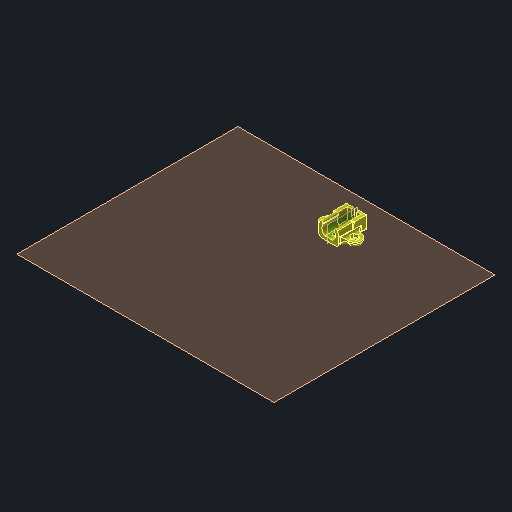
# Autodesk Inventor part: MScIR_WingedMotorHolder-tightened
Saved by Autodesk Inventor 2026.1 (Build 301233020, 233B)
## iProperties
Created: 2018-10-10
Part Number: MScIR_WingedMotorHolder-tightened
Material: ABS Plastic
Document SubType Name: Modeling
Designer: mja502
Density: 1.06 g/cm^3
Appearance: Smooth - White
mountWingsHoleSpacing: 25,200 mm
Author: mja502
Autodesk Inventor part; units mm, degrees
ref_plane "YZ Plane" through (0, 0, 0) normal (1, 0, 0) x (0, 1, 0)
sketch "Body  Clip Bulk OL" plane through (0, 0, 0) normal (0, 0, 1) x (1, 0, 0)
  line L0 (-3.5, 3) -> (3.5, 3)
  line L1 (0, 0) -> (0, 19.508) construction
  line L2 (-6, 8) -> (6, 8) construction
  line L3 (-3.5, 13) -> (3.5, 13)
  arc A0 (-3.5, 13) -> (-3.5, 3) centre (0.25, 8) ccw
  arc A1 (3.5, 3) -> (3.5, 13) centre (-0.25, 8) ccw
  line L4 (4.3935, 16) -> (-4.3935, 16)
  arc A2 (-4.3935, 16) -> (-9, 8) centre (0.25, 8) ccw
  arc A3 (9, 8) -> (4.3935, 16) centre (-0.25, 8) ccw
  line L5 (-9, 8) -> (-9, 0)
  line L6 (9, 8) -> (9, 0)
  line L7 (-9, 0) -> (9, 0)
  point P0 (0, 0)
  point P1 (0, 3)
  point P2 (0, 8)
  point P3 (0, 13)
  point P4 (0, 16)
  dimension "d1" = 7
  dimension "d3" = 12
  dimension "d4" = 5
  dimension "d5" = 10
  dimension "d6" = 3
  dimension "d8" = 3
  dimension "d9" = 18
  constraints: 16 end point, 10 point on circle, 5 midpoint, 4 centre point, 4 horizontal, 4 point on line, 3 vertical, 1 coincident, 1 parallel, 1 tangent
  measures "d1" distance of L0.start L0.end
  measures "d3" distance of L2.start L2.end
  measures "d4" distance between parallel lines of L0 L2
  measures "d5" distance between parallel lines of L0 L3
  measures "d6" distance between parallel lines of L3 L4
  measures "d8" distance from line of point (0, 0) L0
  measures "d9" distance of L5.end L6.end
extrude "Body Clip Bulk" add sketch "Body  Clip Bulk OL" along normal blind 13.8
fillet "Clip Bottom Fillet" radius 2 2 edges at (-9, 0, 6.9) (9, 0, 6.9)
ref_plane "BC Midplane" through (-3.5, 8, 0) normal (0, 1, 0) x (1, 0, 0)
sketch "BC Top Cut OL" plane through (0.0033, 16, 0) normal (0, 1, 0) x (-1, 0, 0)
  line L0 (-5.1967, 13.8) -> (5.2033, 13.8)
  line L1 (5.2033, 13.8) -> (5.2033, 0)
  line L2 (5.2033, 0) -> (-5.1967, 0)
  line L3 (-5.1967, 0) -> (-5.1967, 13.8)
  point P0 (0.0033, 0)
  point P1 (0.0033, 0)
  dimension "d13" = 10.4
  dimension "d14" = 13.8
  constraints: 8 end point, 2 parallel, 1 coincident, 1 horizontal, 1 midpoint, 1 perpendicular
  measures "d13" distance of L0.start L0.end
  measures "d14" distance of L0.end L1.end
extrude "BC Top Cut" cut sketch "BC Top Cut OL" against normal up to surface (8 mm away)
fillet "BC Top Edge Fillets" radius 1.4 2 edges at (5.2, 15.474, 6.9) (-5.2, 15.474, 6.9)
sketch "BC Removal Slot OL" plane through (-3.5, 3, 0) normal (0, 1, 0) x (1, 0, 0)
  line L0 (3.5, 0) -> (3.5, -13.8) construction
  line L1 (7, -13.8) -> (0, -13.8) construction
  line L2 (7, 0) -> (7, -13.8) construction
  line L3 (7, -6.9) -> (0, -6.9) construction
  line L4 (0, 0) -> (0, -13.8) construction
  line L5 (3.5, -5.9) -> (3.5, -7.9) construction
  line L6 (1.5, -5.9) -> (1.5, -7.9)
  line L7 (5.5, -7.9) -> (5.5, -5.9)
  arc A0 (5.5, -5.9) -> (1.5, -5.9) centre (3.5, -5.9) ccw
  arc A1 (1.5, -7.9) -> (5.5, -7.9) centre (3.5, -7.9) ccw
  point P0 (3.5, -6.9)
  dimension "d79" = 6
  dimension "d80" = 4
  constraints: 12 end point, 5 midpoint, 4 point on circle, 4 tangent, 2 centre point, 1 parallel, 1 point on line
  measures "d80" distance between parallel lines of L6 L7
extrude "BC Removal Slot" cut sketch "BC Removal Slot OL" against normal through all
sketch "FS Floor Bulk OL" plane through (0, 0, 0) normal (0, 0, 1) x (1, 0, 0)
  line L0 (-9, 0) -> (9, 0)
  line L1 (9, 0) -> (9, 2.6)
  line L2 (9, 2.6) -> (-9, 2.6)
  line L3 (-9, 2.6) -> (-9, 0)
  line L4 (-7, 0) -> (7, 0) projected
  point P0 (0, 0)
  point P1 (0, 0)
  dimension "d19" = 18
  dimension "d20" = 2.6
  constraints: 8 end point, 2 midpoint, 2 parallel, 1 horizontal, 1 perpendicular
  measures "d19" distance of L0.start L0.end
  measures "d20" distance of L2.end L0.start
extrude "FS Floor Bulk" add sketch "FS Floor Bulk OL" against normal blind 11.2
fillet "FS Bottom Fillet" radius 3 2 edges at (9, 0, -5.6) (-9, 0, -5.6)
sketch "FS Walls OL" plane through (-3.5, 2.6, 4.5) normal (0, 1, 0) x (1, 0, 0)
  line L0 (3.5, 4.5) -> (3.5, 19.7596) construction
  line L1 (-5.5, 4.5) -> (-2.5, 4.5)
  line L2 (-2.5, 4.5) -> (-2.5, 13.7)
  line L3 (-2.5, 13.7) -> (1.3, 13.7)
  line L4 (1.3, 13.7) -> (1.3, 15.7)
  line L5 (1.3, 15.7) -> (-5.5, 15.7)
  line L6 (-5.5, 15.7) -> (-5.5, 4.5)
  line L7 (12.5, 4.5) -> (9.5, 4.5)
  line L8 (9.5, 4.5) -> (9.5, 13.7)
  line L9 (9.5, 13.7) -> (5.7, 13.7)
  line L10 (5.7, 13.7) -> (5.7, 15.7)
  line L11 (5.7, 15.7) -> (12.5, 15.7)
  line L12 (12.5, 15.7) -> (12.5, 4.5)
  dimension "d24" = 6.8
  dimension "d25" = 2
  dimension "d26" = 3
  dimension "d27" = 9.2
  dimension "d28" = 11.2
  dimension "d32" = 9
  constraints: 26 end point, 6 symmetric about line, 5 perpendicular, 1 horizontal, 1 vertical
  measures "d24" distance of L4.end L5.end
  measures "d25" distance of L3.end L4.end
  measures "d26" distance of L1.start L1.end
  measures "d27" distance of L1.end L2.end
  measures "d28" vertical distance of L0.start L5.end
  measures "d32" distance of L0.start L1.start
extrude "FS Walls" add sketch "FS Walls OL" along normal blind 10.4
sketch "FS Shaft Slot Seat OL" plane through (0, 0, -11.2) normal (0, 0, -1) x (-1, 0, 0)
  line L0 (0, 0) -> (0, 7.8) construction
  circle A0 centre (0, 7.8) radius 2.2
  line L1 (-2.2, 7.8) -> (-2.2, 2.6)
  line L2 (-2.2, 2.6) -> (2.2, 2.6)
  line L3 (2.2, 2.6) -> (2.2, 7.8)
  dimension "d33" = 7.8
  dimension "d34" = 4.4
  dimension "d35" = 5.2
  dimension "d36" = 4.4
  constraints: 8 end point, 2 coincident, 2 perpendicular, 2 point on circle, 2 vertical, 1 centre point, 1 parallel
  measures "d33" distance of L0.start L0.end
  measures "d34" diameter of A0
  measures "d35" distance of L2.end L3.end
  measures "d36" distance of L1.end L2.end
extrude "FS Front Shaft Seat" add sketch "FS Shaft Slot Seat OL" against normal blind 2 contours L3 L2 L1 A0
sketch "FS Pillars OL" plane through (-3.5, 3, 13.8) normal (0, 1, 0) x (1, 0, 0)
  line L0 (8.9, 13.8) -> (9.5, 13.8)
  line L1 (9.5, 13.8) -> (9.5, 15.7)
  line L2 (9.5, 15.7) -> (8.9, 15.7)
  line L3 (8.9, 15.7) -> (8.9, 13.8)
  line L4 (-2.5, 16.1) -> (-1.9, 16.1)
  line L5 (-1.9, 16.1) -> (-1.9, 20)
  line L6 (-1.9, 20) -> (-2.5, 20)
  line L7 (-2.5, 20) -> (-2.5, 16.1)
  point P0 (3.5, 13.8)
  dimension "d39" = 0.6
  dimension "d40" = 1.9
  dimension "d41" = 6
  dimension "d42" = 0
  dimension "d43" = 0.6
  dimension "d44" = 3.9
  dimension "d46" = 6
  dimension "d47" = 2.3
  constraints: 16 end point, 4 parallel, 2 horizontal, 2 perpendicular
  measures "d39" distance of L2.end L1.end
  measures "d40" distance of L1.end L0.end
  measures "d41" distance of point (3.5, 13.8) L0.end
  measures "d42" distance from line of point (3.5, 13.8) L0
  measures "d43" distance of L6.end L5.end
  measures "d44" distance of L5.end L4.end
  measures "d46" horizontal distance of point (3.5, 13.8) L4.start
  measures "d47" distance from line of point (3.5, 13.8) L4
extrude "FS Pillars" [suppressed]
sketch "Sketch9" plane through (9, 8, 13.8) normal (1, 0, 0) x (0, 0, -1)
  line L0 (13.8, -6) -> (13.8, -5.4) projected
  line L1 (13.8, -5.4) -> (3.1659, 5.2341)
  line L2 (13.8, 5.2341) -> (0, 5.2341) projected
  line L3 (13.8, -5.4) -> (28.8388, -5.4) construction
  line L4 (13.8, -5.4) -> (13.8, 5.2341)
  point P0 (13.8, -8)
  dimension "d50" = 135
  constraints: 6 end point, 1 equal length, 1 horizontal, 1 point on line
  measures "d50" angle of L3 L1
extrude "BC 45deg cut" [suppressed]
ref_plane "Encoder Section Plane" through (0, 0, 13.8) normal (0, 0, 1) x (1, 0, 0)
sketch "Sketch10" plane through (0, 0, 13.8) normal (0, 0, 1) x (1, 0, 0)
  line L0 (-9, 2) -> (9, 2)
  line L1 (9, 2) -> (9, 0)
  line L2 (9, 0) -> (-9, 0)
  line L3 (-9, 0) -> (-9, 2)
  point P0 (0, 0)
  point P1 (0, 0)
  dimension "d54" = 2
  dimension "d55" = 18
  constraints: 8 end point, 2 parallel, 1 coincident, 1 horizontal, 1 midpoint, 1 perpendicular
  measures "d54" distance of L0.end L1.end
  measures "d55" distance of L1.end L2.end
extrude "ES Floor" [suppressed]
fillet "ES Bottom Fillet" [suppressed]
sketch "ES walls OL" plane through (-8.8284, 2, 13.8) normal (0, 1, 0) x (1, 0, 0)
  line L0 (-0.1716, 0) -> (-0.1716, -9.1)
  line L1 (-0.1716, -9.1) -> (17.8284, -9.1)
  line L2 (17.8284, -9.1) -> (17.8284, 0)
  line L3 (17.8284, 0) -> (15.5284, 0)
  line L4 (15.5284, 0) -> (15.5284, -7.1)
  line L5 (15.5284, -7.1) -> (2.1284, -7.1)
  line L6 (2.1284, -7.1) -> (2.1284, 0)
  line L7 (2.1284, 0) -> (-0.1716, 0)
  point P0 (8.8284, 13.8)
  dimension "d59" = 2.3
  dimension "d60" = 2
  dimension "d61" = 9.1
  dimension "d62" = 18
  constraints: 16 end point, 6 perpendicular, 2 equal length, 1 coincident, 1 horizontal, 1 point on line, 1 vertical
  measures "d59" distance between parallel lines of L2 L4
  measures "d60" distance between parallel lines of L1 L5
  measures "d61" distance of L1.end L2.end
  measures "d62" distance of L0.end L1.end
extrude "ES Walls" [suppressed]
sketch "ES Slot ol" plane through (-6.7, 2, 13.8) normal (0, 1, 0) x (1, 0, 0)
  line L0 (13.6, -1.8) -> (-0.2, -1.8)
  line L1 (-0.2, -1.8) -> (-0.2, -5.2)
  line L2 (-0.2, -5.2) -> (13.6, -5.2)
  line L3 (13.6, -5.2) -> (13.6, -1.8)
  line L4 (10.2, 0) -> (3.2, 0) construction
  line L5 (6.7, 0) -> (6.7, -5.8979) construction
  line L6 (13.6, -3.5) -> (-0.2, -3.5) construction
  point P0 (6.7, 13.8)
  point P1 (6.7, -1.8)
  dimension "d65" = 13.8
  dimension "d66" = 3.4
  dimension "d67" = 3.5
  constraints: 12 end point, 4 midpoint, 2 parallel, 1 horizontal, 1 perpendicular, 1 point on line, 1 vertical
  measures "d65" distance of L1.end L2.end
  measures "d66" distance of L0.end L1.end
  measures "d67" distance between parallel lines of L4 L6
extrude "ES Slot" [suppressed]
sketch "Sketch13" plane through (0, 0, 22.9) normal (0, 0, 1) x (1, 0, 0)
  line L0 (0, 0) -> (0, 7) construction
  line L1 (-6.1716, 0) -> (6.1716, 0) construction
  circle A0 centre (0, 7) radius 4.45
  line L2 (4.45, 7) -> (4.45, 13)
  line L3 (4.45, 13) -> (-4.45, 13)
  line L4 (-9, 13) -> (9, 13) construction
  line L5 (-4.45, 13) -> (-4.45, 7)
  point P0 (0, 0)
  dimension "d70" = 7
  dimension "d71" = 8.9
  constraints: 8 end point, 3 vertical, 2 point on circle, 2 tangent, 1 centre point, 1 coincident, 1 collinear, 1 midpoint, 1 perpendicular
  measures "d70" distance of L0.start L0.end
  measures "d71" diameter of A0
extrude "ES Rear Cutaway" [suppressed]
fillet "ES Merge Fillet" radius 0.95 4 edges at (-7.627, 12.7855, 0) (-8.7006, 10.3345, 0) (7.627, 12.7855, 0) (8.7006, 10.3345, 0)
fillet "ES Cutaway Fille" [suppressed]
sketch "Sketch16" plane through (-6.7, 2, 15.6) normal (0, 0, 1) x (1, 0, 0)
  arc A0 (-0.2, -1.9102) -> (0.5284, -2) centre (0.5284, 1) ccw projected
  line L0 (12.8716, -2) -> (0.5284, -2) projected
  arc A1 (12.8716, -2) -> (13.6, -1.9102) centre (12.8716, 1) ccw projected
  line L1 (13.6, 11) -> (13.6, -1.9102) projected
  line L2 (13.4, 11) -> (13.6, 11) projected
  line L3 (13.4, 0) -> (13.4, 11) projected
  line L4 (0, 0) -> (13.4, 0) projected
  line L5 (0, 11) -> (0, 0) projected
  line L6 (-0.2, 11) -> (0, 11) projected
  line L7 (-0.2, -1.9102) -> (-0.2, 11) projected
  point P0 (6.7, -2)
  point P1 (0, -1.9531)
  point P2 (13.4, -1.9531)
  constraints: 2 point on circle
extrude "ES Pins Undercut" [suppressed]
chamfer "ES Pins Undercut CHamfer" [suppressed]
ref_plane "Midplane" through (0, 0, 2.8) normal (0, 0, -1) x (-1, 0, 0)
sketch "Sketch17" plane through (-6, 0, -11.2) normal (0, -1, 0) x (1, 0, 0)
  line L0 (26.68, 14) -> (-18.68, 14) construction
  line L1 (6, 14) -> (6, 11.2) construction
  circle A0 centre (18.6, 14) radius 1.6 construction
  circle A1 centre (-6.6, 14) radius 1.6
  line L2 (-6.6, 8.4) -> (-6.6, 19.6) construction
  line L3 (-6.6, 14) -> (-12.2, 14) construction
  line L4 (-3, 0) -> (-3, 11.2) construction
  line L5 (-3, 25) -> (-3, 34.1) construction
  arc A2 (-6.6, 19.6) -> (-6.6, 8.4) centre (-6.6, 14) ccw
  arc A3 (-3, 4.8) -> (-6.6, 8.4) centre (-6.6, 4.8) ccw
  arc A4 (-6.6, 19.6) -> (-3, 23.2) centre (-6.6, 23.2) ccw
  line L6 (-3, 4.8) -> (-3, 23.2)
  dimension "d88" = 3.2
  dimension "d89" = 25.2
  dimension "d90" = 11.2
  dimension "d91" = 5.6
  constraints: 8 end point, 7 point on circle, 5 centre point, 5 point on line, 4 tangent, 3 vertical, 1 equal radius, 1 horizontal, 1 midpoint, 1 symmetric about line
  measures "d88" diameter of A0
  measures "d89" distance of L3.start A0.centre
  measures "d90" distance of L2.start L2.end
  measures "d91" distance of L3.start L3.end
extrude "Wing Bulk" add sketch "Sketch17" against normal blind 4.4
sketch "Sketch18" plane through (-9, 0, 12) normal (1, 0, 0) x (0, 0, -1)
  line L0 (0, 3) -> (12, 3) projected
  line L1 (0, 0) -> (0, 3) projected
  line L2 (0, 0) -> (18.4, 0) projected
  line L3 (18.4, 0) -> (18.4, 2.6) projected
  line L4 (18.4, 2.6) -> (12, 2.6) projected
  line L5 (12, 2.6) -> (12, 3) projected
  point P0 (12, 0)
extrude "Wing Underside Merge" add sketch "Sketch18" along normal up to surface (7 mm away)
fillet "Wing UNderside Fillet" radius 3 3 edges at (-18.2, 0, 2.8) (-10.0544, 0, -3.8544) (-10.0544, 0, 9.4544)
sketch "Sketch19" plane through (-6, 4.4, -11.2) normal (0, 1, 0) x (1, 0, 0)
  circle A0 centre (-6.6, -14) radius 1.6 projected
  line L0 (-6.6, -10.6514) -> (-3.7, -12.3257)
  line L1 (-3.7, -12.3257) -> (-3.7, -15.6743)
  line L2 (-3.7, -15.6743) -> (-6.6, -17.3486)
  line L3 (-6.6, -17.3486) -> (-9.5, -15.6743)
  line L4 (-9.5, -15.6743) -> (-9.5, -12.3257)
  line L5 (-9.5, -12.3257) -> (-6.6, -10.6514)
  line L6 (-17.6406, -14) -> (20.4437, -14) construction
  point P0 (6, -11.2)
  dimension "d98" = 5.8
  constraints: 12 end point, 1 coincident, 1 perpendicular, 13 other
  measures "d98" distance between parallel lines of L4 L1
extrude "Wing Nut Cut" cut sketch "Sketch19" against normal blind 2.4
mirror "Wing Mirror" about plane through (0, 0, 0) normal (1, 0, 0) of "Wing Bulk", "Wing Underside Merge", "Wing UNderside Fillet", "Wing Nut Cut"
fillet "Wings Top Fillet" radius 3 2 edges at (-9, 4.4, 2.8) (9, 4.4, 2.8)
sketch "Sketch20" plane through (6.7, 2, 19) normal (0, 0, -1) x (-1, 0, 0)
  line L0 (-0.2, 11) -> (-0.0716, 11) projected
  line L1 (-0.2, -1.9102) -> (-0.2, 11) projected
  arc A0 (-0.2, -1.9102) -> (0.5284, -2) centre (0.5284, 1) ccw projected
  line L2 (12.8716, -2) -> (0.5284, -2) projected
  arc A1 (12.8716, -2) -> (13.6, -1.9102) centre (12.8716, 1) ccw projected
  line L3 (13.6, -1.9102) -> (13.6, 11) projected
  line L4 (13.4716, 11) -> (13.6, 11) projected
  line L5 (13.4, 0) -> (13.4, 10.9995) projected
  line L6 (0, 0) -> (13.4, 0) projected
  line L7 (0, 10.9995) -> (0, 0) projected
  point P0 (6.7, -2)
  constraints: 2 other
extrude "Slot Enlarging" [suppressed]
sketch "Sketch21" plane through (-6, 0, 13.8) normal (0, -1, 0) x (1, 0, 0)
  arc A0 (4, -7.9) -> (8, -7.9) centre (6, -7.9) ccw projected
  line L0 (8, -5.9) -> (8, -7.9) projected
  arc A1 (8, -5.9) -> (4, -5.9) centre (6, -5.9) ccw projected
  line L1 (4, -7.9) -> (4, -5.9) projected
  point P0 (6, -13.8)
extrude "Extrusion18" cut sketch "Sketch21" against normal through all
ref_plane "Work Plane5" through (0, 2.6, -9.2) normal (-1, 0, 0) x (0, 0, 1)
ref_plane "Work Plane6" through (-15.0139, 0, 63.8653) normal (0, 1, 0) x (-1, 0, 0)
equation "\"d1\" = mo_mBodyFlatsWidth + mo_bcFlatWidthExtra"
equation "\"d3\" = mo_mBodyDiam + mo_bcBodyExtra"
equation "\"d4\" = 0.5 * mo_bcHeightExtra + 0.5 * mo_mBodyFlatsDiam"
equation "\"d5\" = mo_mBodyFlatsDiam + mo_bcHeightExtra"
equation "\"d6\" = mo_bcWallThickness"
equation "\"d8\" = mo_bcWallThickness"
equation "\"d9\" = mo_bcTotalWidth"
equation "\"d10\" = mo_bcLength"
equation "\"d12\" = mo_bcBottomFillet"
equation "\"d13\" = mo_bcTopCutWidth"
equation "\"d14\" = mo_bcLength"
equation "\"d15\" = mo_mBodyLength"
equation "\"d18\" = mo_bcOpeningFillet"
equation "\"d19\" = mo_fsTotalWidth"
equation "\"d20\" = mo_fsFloorDepth"
equation "\"d23\" = mo_fsBottomFillet"
equation "\"d24\" = 0.5 * mo_fsTotalWidth - 0.5 * mo_fsShaftSlotWidth"
equation "\"d25\" = mo_fsFrontThickness"
equation "\"d26\" = mo_fsWallThickness"
equation "\"d32\" = 0.5 * mo_fsTotalWidth"
equation "\"d30\" = mo_fsTotalHeight - mo_fsFloorDepth"
equation "\"d33\" = 0.5 * mo_mGbHeight + mo_fsFloorDepth + 0.5 * mo_fsShaftSlotClearance"
equation "\"d34\" = mo_fsShaftSlotWidth"
equation "\"d35\" = 0.5 * mo_mGbHeight + 0.5 * mo_fsShaftSlotClearance"
equation "\"d36\" = mo_fsShaftSlotWidth"
equation "\"d37\" = mo_fsFrontThickness"
equation "\"d39\" = mo_fsPillarDepth"
equation "\"d40\" = mo_fsThinPillarWidth"
equation "\"d41\" = 0.5 * mo_fsTotalWidth - mo_fsWallThickness"
equation "\"d43\" = mo_fsPillarDepth"
equation "\"d44\" = mo_fsThickPillarWidth"
equation "\"d46\" = 0.5 * mo_fsTotalWidth - mo_fsWallThickness"
equation "\"d47\" = mo_fsThickPillarOffset"
equation "\"d48\" = mo_fsPillarHeight"
equation "\"d51\" = mo_fsPillarHeight"
equation "\"d54\" = mo_esFloorDepth"
equation "\"d55\" = mo_esTotalWidth"
equation "\"d56\" = mo_esTotalLength"
equation "\"d58\" = mo_esBottomFillet"
equation "\"d59\" = mo_esWallThickness"
equation "\"d60\" = mo_esRearWallThickness"
equation "\"d61\" = mo_esTotalLength"
equation "\"d62\" = mo_esTotalWidth"
equation "\"d63\" = mo_esTotalHeight - mo_esFloorDepth"
equation "\"d65\" = mo_esSlotLength"
equation "\"d66\" = mo_esSlotWidth"
equation "\"d67\" = mo_esSlotOffset"
equation "\"d70\" = mo_esRearCutawayHeight + mo_esFloorDepth"
equation "\"d71\" = mo_esRearCutawayDiam"
equation "\"d75\" = mo_esRearCutawayFillet"
equation "\"mo_mBodyDiam\" = 12"
equation "\"mo_mBodyFlatsDiam\" = 10"
equation "\"mo_mBodyLength\" = 15"
equation "\"mo_mShaftDiam\" = 3"
equation "\"mo_mShaftLength\" = 11"
equation "\"mo_mShaftFlatDiam\" = 2.5"
equation "\"mo_mGb_shaftBaseDiam\" = 4"
equation "\"mo_mGb_shaftBaseThickness\" = 1"
equation "\"mo_mEncTotalHeight\" = 16.6"
equation "\"mo_mEncTotalWidth\" = 12.6"
equation "\"mo_mEncPinsOffset\" = 3.5"
equation "\"mo_mGbPlateSpacingFront\" = 4.3"
equation "\"mo_mEncTotalExtent\" = 5.4"
equation "\"mo_mGbPlateSpacingRear\" = 2.3"
equation "\"mo_mGbLength\" = 9"
equation "\"mo_mGbWidth\" = 12"
equation "\"mo_mGbPlateThickness\" = 0.8"
equation "\"mo_mBodyFlatsWidth\" = 7"
equation "\"mo_bcTopCutWidth\" = 10.4"
equation "\"mo_bcHeightExtra\" = 0"
equation "\"mo_bcFlatWidthExtra\" = 0"
equation "\"mo_bcLength\" = 13.8"
equation "\"mo_bcBodyExtra\" = 0"
equation "\"mo_bcWallThickness\" = 3"
equation "\"mo_bcBottomFillet\" = 2"
equation "\"mo_bcOpeningFillet\" = 1.4"
equation "\"mo_bcTopOverlap\" = 0.8"
equation "\"mo_bcTotalWidth\" = 18"
equation "\"mo_fsWallThickness\" = mo_bcWallThickness - mo_fsSideClearance"
equation "\"mo_fsFrontClearance\" = 0.6"
equation "\"mo_fsSideClearance\" = 0"
equation "\"mo_fsFloorDepth\" = mo_bcWallThickness - mo_fsFloorReduction"
equation "\"mo_fsTotalWidth\" = 18"
equation "\"mo_fsTotalHeight\" = mo_fsFloorDepth + mo_mGbHeight + mo_fsFloorReduction"
equation "\"mo_fsFrontThickness\" = 2"
equation "\"mo_fsTotalLength\" = mo_fsFrontClearance + mo_mGbLength + mo_fsFrontThickness"
equation "\"mo_fsBottomFillet\" = 3"
equation "\"mo_fsPlateClearance\" = 0.2"
equation "\"mo_fsStartOffset\" = mo_mGbPlateThickness"
equation "\"mo_fsShaftSlotWidth\" = mo_mGb_shaftBaseDiam + mo_fsShaftSlotClearance"
equation "\"mo_fsPillarDepth\" = 0.6"
equation "\"mo_fsThinPillarOffset\" = 0"
equation "\"mo_fsThickPillarWidth\" = 3.9"
equation "\"mo_fsThinPillarWidth\" = 1.9"
equation "\"mo_fsThickPillarOffset\" = 2.3"
equation "\"mo_fsPillarHeight\" = 3"
equation "\"mo_fsFloorReduction\" = 0.4"
equation "\"mo_fsShaftSlotClearance\" = 0.4"
equation "\"mo_mEncMagnetThickness\" = 2"
equation "\"mo_mEncMagnetDiam\" = 7.7"
equation "\"mo_mEncTotalLength\" = 6.5"
equation "\"mo_mEncPinsThickness\" = 2.2"
equation "\"mo_esSlotPinsClearance\" = 0.6"
equation "\"mo_esSlotWidth\" = 3.4"
equation "\"mo_esSlotOffset\" = mo_mEncPinsOffset"
equation "\"mo_esSlotLength\" = 13.8"
equation "\"mo_esRearMagnetClearance\" = 0.6"
equation "\"mo_esRearClearance\" = 2.6"
equation "\"mo_esRearWallThickness\" = 2"
equation "\"mo_esSideClearance\" = 0.4"
equation "\"mo_esFloorDepth\" = 2"
equation "\"mo_esTotalHeight\" = mo_fsTotalHeight"
equation "\"mo_esTotalWidth\" = mo_fsTotalWidth"
equation "\"d53\" = mo_bcLength"
equation "\"mo_esWallThickness\" = 2.3"
equation "\"mo_esBottomFillet\" = 3"
equation "\"mo_esTotalLength\" = 9.1"
equation "\"mo_esRearCutawayDiam\" = 8.9"
equation "\"mo_esRearCutawayHeight\" = 5"
equation "\"mo_esTopFillet\" = 2.2"
equation "\"mo_esRearCutawayFillet\" = 3"
equation "\"mo_esMergeFillet\" = 1.25"
equation "\"mo_bcRemovalSlotLength\" = 6"
equation "\"mo_bcRemovalSlotWidth\" = 4"
equation "\"mo_esPinsUndercutChamfer\" = 2"
equation "\"mo_esPinsUndercut\" = 1.8"
equation "\"mo_bcMatingSurfaceCompensation\" = 0.4"
equation "\"mo_bcRemovalSlotRearOffset\" = 15"
equation "\"mo_pcbLedLeftOffset\" = 2.4"
equation "\"mo_phrClipWidth\" = 5"
equation "\"mo_phrConnClearance\" = 0.4"
equation "\"mo_phrClipLength\" = 7.6"
equation "\"mo_phFlatDepth\" = 3"
equation "\"mo_phrShelfOverlapLeft\" = 0.5"
equation "\"mo_phrShelfOverlapRight\" = 0.5"
equation "\"mo_phrClipSlotLength\" = 5.2"
equation "\"mo_phrClipSlotWidth\" = 2"
equation "\"mo_phWallThickness\" = 2"
equation "\"mo_phFlatLength\" = 34.5"
equation "\"mo_phBoardClearance\" = 0.2"
equation "\"mo_pcbDipOffsetRear\" = 2.9"
equation "\"mo_pcbWidth\" = 20.4"
equation "\"mo_pcbDipOffsetSide\" = 2.8"
equation "\"mo_pcbDipWidth\" = 6.2"
equation "\"mo_pcbConnRightOffset\" = 2.4"
equation "\"mo_pcbBoardThickness\" = 1.55"
equation "\"mo_pcbConnWidth\" = 4.3"
equation "\"mo_pcbJackHoleDiameter\" = 4.9"
equation "\"mo_pcbFrontJackFrontOffset\" = 5.2"
equation "\"mo_pcbConnHeight\" = 3.2"
equation "\"mo_pcbHeight\" = 7.2"
equation "\"mo_pcbDipLength\" = 6.2"
equation "\"mo_pcbLedFrontOffset\" = 5.6"
equation "\"mo_pcbRearJackFrontOffset\" = 12.9"
equation "\"mo_flTongueSideClearance\" = 0.1"
equation "\"mo_flToothInnerBaseFillet\" = 2"
equation "\"mo_flToothClearance\" = 0.2"
equation "\"mo_rlToothRearOffset\" = 2"
equation "\"mo_flTongueFrontClearance\" = 0.4"
equation "\"mo_rlTotalLength\" = 16"
equation "\"mo_rlToothInnerBaseFillet\" = 2"
equation "\"mo_flToothTipFillet\" = 0.6"
equation "\"mo_esShaftSlotLength\" = 7"
equation "\"mo_flToothBaseWidth\" = 3"
equation "\"mo_flToothDepth\" = 3"
equation "\"mo_esShaftSlotWidth\" = 1.6"
equation "\"mo_flExtraLength\" = 0.6"
equation "\"mo_flToothAngle\" = 0.01deg"
equation "\"mo_flTotalLength\" = 18.5"
equation "\"mo_flToothFrontOffset\" = 5"
equation "\"mo_mGbHeight\" = 10"
body "Solid1"
